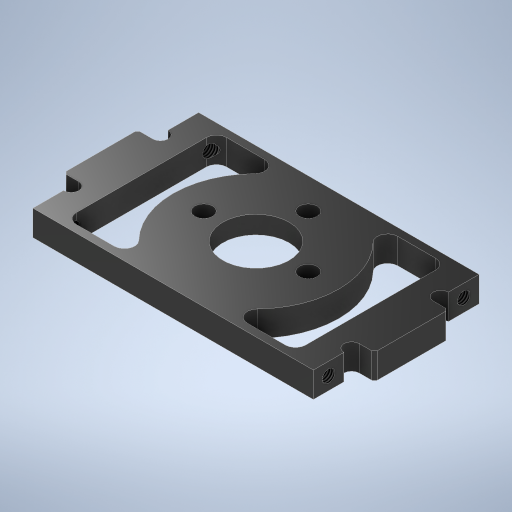
# Autodesk Inventor part: HeadHornFrame
Saved by Autodesk Inventor 2024.2 (Build 282272000, 272)
## iProperties
Created: 2024-01-28
Part Number: HeadHornFrame
Material: Aluminum 7075
Document SubType Name: Modeling
Designer: Masato Kubotera
Density: 2.81 g/cm^3
Appearance: Glossy - Black
Vendor: meviy
Mass: 14.5344 g
Surface Area: 47.0549 cm^2
Volume: 5.17237 cm^3
Author: Masato Kubotera
Autodesk Inventor part; units mm, degrees
ref_plane "YZ Plane" through (0, 0, 0) normal (1, 0, 0) x (0, 1, 0)
ref_plane "XZ Plane" through (0, 0, 0) normal (0, 1, 0) x (-1, 0, 0)
ref_plane "XY Plane" through (0, 0, 0) normal (0, 0, 1) x (1, 0, 0)
sketch "Sketch1" plane through (0, 0, 0) normal (0, 0, 1) x (1, 0, 0)
  line L0 (-16.25, 0) -> (16.25, 0)
  circle A0 centre (0, 0) radius 14.75 construction
  circle A1 centre (0, 0) radius 12.5 construction
  circle A2 centre (0, 0) radius 14.8
  line L1 (0, 0) -> (10.4298, 10.4298) construction
  arc A3 (8.7552, 11.9326) -> (11.9326, 8.7552) centre (10.4298, 10.4298) ccw
  arc A4 (-11.9326, 8.7552) -> (-8.7552, 11.9326) centre (-10.4298, 10.4298) ccw
  arc A5 (-8.7552, -11.9326) -> (-11.9326, -8.7552) centre (-10.4298, -10.4298) ccw
  arc A6 (11.9326, -8.7552) -> (8.7552, -11.9326) centre (10.4298, -10.4298) ccw
  line L2 (16.25, 27.5) -> (-16.25, 27.5)
  line L3 (-16.25, 27.5) -> (-16.25, -27.5)
  line L4 (-16.25, -27.5) -> (16.25, -27.5)
  line L5 (16.25, -27.5) -> (16.25, 27.5)
  line L6 (16.25, 27.5) -> (-16.25, -27.5) construction
  line L7 (-16.25, 27.5) -> (16.25, -27.5) construction
  line L8 (-7.25, -27.5) -> (-7.25, -30.5)
  line L9 (-7.25, -30.5) -> (7.25, -30.5)
  line L10 (7.25, -30.5) -> (7.25, -27.5)
  line L11 (0, -27.5) -> (0, 27.5) construction
  arc A7 (-7.25, -27.5) -> (-10.25, -27.5) centre (-8.75, -27.5) ccw
  arc A8 (10.25, -27.5) -> (7.25, -27.5) centre (8.75, -27.5) ccw
  line L12 (-13.25, -27.5) -> (-13.25, -21.5) construction
  line L13 (13.25, -27.5) -> (13.25, -21.5) construction
  line L14 (-7.25, 27.5) -> (-7.25, 30.5)
  line L15 (-7.25, 30.5) -> (7.25, 30.5)
  line L16 (7.25, 30.5) -> (7.25, 27.5)
  arc A9 (-10.25, 27.5) -> (-7.25, 27.5) centre (-8.75, 27.5) ccw
  arc A10 (7.25, 27.5) -> (10.25, 27.5) centre (8.75, 27.5) ccw
  line L17 (-13.25, 27.5) -> (-13.25, 21.5) construction
  line L18 (13.25, 27.5) -> (13.25, 21.5) construction
  line L19 (14.75, 22.5) -> (-14.75, 22.5)
  line L20 (-14.75, 22.5) -> (-14.75, 6.8191)
  arc A11 (14.75, 6.8191) -> (-14.75, 6.8191) centre (0, 0) ccw
  line L21 (14.75, 22.5) -> (14.75, 6.8191)
  point P0 (10.25, 0)
  point P1 (0, 10.25)
  point P2 (-10.25, 0)
  point P3 (0, -10.25)
  point P4 (16.25, 0)
  point P5 (10.25, 27.5)
  point P6 (-10.25, 27.5)
  point P7 (-14.8, 0)
  point P8 (14.8, 0)
  point P9 (7.25, 27.5)
  point P10 (-7.25, 27.5)
  dimension "d11" = 29.5
  dimension "d9" = 360
  dimension "d10" = 20.5
  dimension "d12" = 25
  dimension "d13" = 0.05
  dimension "d14" = 360
  dimension "d19" = 32.5
  dimension "d20" = 55
  dimension "d21" = 1.5
  dimension "d23" = 3
  dimension "d24" = 6
  dimension "d25" = 6
  dimension "d56" = 3
  dimension "d57" = 5
  constraints: 45 end point, 20 point on circle, 20 symmetric about line, 11 centre point, 8 midpoint, 7 coincident, 6 point on line, 4 horizontal, 4 vertical, 2 parallel, 2 tangent, 1 concentric, 1 perpendicular, 29 other
  measures "d10" distance of point (-10.25, 0) point (10.25, 0)
  measures "d12" diameter of A1
  measures "d19" distance of L4.end L3.end
  measures "d20" distance of L3.end L2.end
  measures "d21" radius of A7
  measures "d23" distance of L8.start L8.end
  measures "d24" distance of L12.start L12.end
  measures "d25" distance of A7.end L3.end
  measures "d56" diameter of L21 L18
  measures "d57" distance between parallel lines of L2 L19
extrude "Extrusion1" add sketch "Sketch1" along normal blind 5 contours A2 L0 L3 L2 A9 A10 L5 | L0 A2 A4 A3 | A3 A2 | A2 A4 | L2 L14 L15 L16
extrude "Extrusion2" cut sketch "Sketch1" along normal blind 1.5 contours L0 A2 A4 A3
fillet "Fillet1" radius 2 8 edges at (-8.7552, 11.9326, 0.75) (-11.9326, 8.7552, 0.75) (11.9326, 8.7552, 0.75) (8.7552, 11.9326, 0.75) (14.75, 22.5, 2.5) (14.75, 6.8191, 2.5) (-14.75, 22.5, 2.5) (-14.75, 6.8191, 2.5)
sketch "Sketch2" plane through (-16.25, 27.5, 0) normal (0, 1, 0) x (-1, 0, 0)
  line L0 (0, 5) -> (-26.5, 5) projected
  line L1 (-6, 5) -> (-32.5, 5) projected
  line L2 (-32.5, 0) -> (0, 0) projected
  line L3 (-32.5, 0) -> (0, 0) projected
  line L4 (-3, 0) -> (-3, 5)
  line L5 (-29.5, 0) -> (-29.5, 5)
  point P0 (-3, 0)
  point P1 (-29.5, 0)
  point P2 (-6, 0)
  point P3 (-26.5, 0)
  point P4 (-29.5, 2.5)
  point P5 (-3, 2.5)
  constraints: 4 end point, 2 midpoint, 2 point on line, 2 vertical
hole "Hole1" at (13.25, 27.5, 2.5) at (-13.25, 27.5, 2.5) direction (0, -1, 0) diameter 2.459 depth 6 thread size "M3x0.5" class "6H" standard "ANSI Metric M Profile"
hole "Hole2" at (0, -10.25, 0) at (-10.25, 0, 0) at (0, 10.25, 0) direction (0, 0, 1) diameter 3.5 end through all
hole "Hole3" at (0, 0, 0) direction (0, 0, 1) diameter 13 end through all
chamfer "Chamfer1" distance 0.5 angle 45 2 edges at (7.25, 30.5, 2.5) (-7.25, 30.5, 2.5)
mirror "Mirror1" about plane through (0, 0, 0) normal (0, 1, 0)
equation "\"d37\" = d24"
equation "\"d44\" = d24"
body "Solid1"
